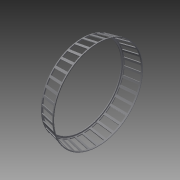
# Autodesk Inventor part: 32912_cage
Saved by Autodesk Inventor 2014 SP2 (Build 180246200, 246)
## iProperties
Created: 2018-11-12
Part Number: 32912_cage
Material: Generic
Catalog Web Link: www.cadenas.de
Description: BT1_001_101_cage-Tapered roller bearings, single row
Vendor: SKF
Document SubType Name: Modeling
Designer: psadmin
Manufacturer: SKF
Mass: 1.044 g
Surface Area: 42.9742 cm^2
Volume: 1.044 cm^3
Density: 1 g/cm^3
Appearance: PSOLRGB-175-175-175
Category: PARTsolutions
Company: SKF
Title: 32912_cage
Author: Cadenas PARTsolutions
Comments: Tapered roller bearings, single row
PSOL_IDENT_0: {$CADENAS_DATA\23d-libs\skf\bearings_units_and_housings\roller_bearings\tapered_roller_bearings\tape
PSOL_IDENT_1: red_roller_bearings_single_row\parts\bt1_001_101_cage.prj},172 {VTYP=3D},{NB=32912_cage},{LINA=32912
PSOL_IDENT_2: _cage},{NN=BT1_001_101_cage},{DATE=14.08.2018 07:35:10},{GEOMDATE=27.06.2018 08:15:48},{VERSION=},{L
PSOL_IDENT_3: INEID=2140},{WBVAR=},{WBNUMERIC=}  {NB=32912_cage},{LINA=32912_cage},{KT=DUMMY},{DESIGNATION=32912},
PSOL_IDENT_4: {DD=60.000},{D=85.000},{T=17.000},{DD1=73.8000},{D1=MIN},{B=17.000},{C=14.000},{C1=MIN},{R12=1.0},{R
PSOL_IDENT_5: 34=1.0},{AA=15.45165},{PITCH=72.347},{DW=5.200},{LW=12.200},{RANGLE=1.600},{ALPHA=12.450},{DDAMAX=67
PSOL_IDENT_6: },{DDAMIN=68.0},{DAMIN=78},{DAMAX=78.0},{DBMIN=81},{CA=3},{CB=3.0},{RA=1.0},{RB=1.0},{LOAD1=53.200},
PSOL_IDENT_7: {LOAD2=75.000},{LOAD3=7.800},{SPEED1=6000},{SPEED2=7000},{EE=0.33},{Y=1.80},{Y0=1.0},{Y1=0},{X1=1},{
PSOL_IDENT_8: X2=0.4},{X0=0.5},{Z=34},{II=1},{R1=0.00000231},{R2=10.9},{S1=0.009},{S2=2},{KZ=6},{KL=0.7},{BF=2},{M
PSOL_IDENT_9: ASS=0.302},{PIM=PIM_BT1_001},{DESIGN=trb1},{HELP=0.000}
NN: BT1_001_101_cage
NT: Tapered roller bearings, single row
NB: 32912_cage
NBSYN: $DESIGNATION._cage
LINA: 32912_cage
DESIGNATION: 32912
DD: 60
D: 85
T: 17
DD1: 73.8
D1: 0
B: 17
C: 14
C1: 0
R12: 1
R34: 1
AA: 15.45165
PITCH: 72.347
DW: 5.2
LW: 12.2
RANGLE: 1.6
ALPHA: 12.45
DDAMAX: 67
DDAMIN: 68
DAMIN: 78
DAMAX: 78
DBMIN: 81
CA: 3
CB: 3
RA: 1
RB: 1
LOAD1: 53.2
LOAD2: 75
LOAD3: 7.8
SPEED1: 6000
SPEED2: 7000
EE: 0.33
Y: 1.8
Y0: 1
Y1: 0
X1: 1
X2: 0.4
X0: 0.5
Z: 34
II: 1
R1: 0.00000231
R2: 10.9
S1: 0.009
S2: 2
KZ: 6
KL: 0.7
BF: 2
MASS: 0.302
PIM: PIM_BT1_001
SUPPLIER: SKF
ARTICLENO: 32912_cage
BOMINFO: 32912_cage
CREATOR: CADENAS GmbH
Autodesk Inventor part; units mm, degrees
sketch "Sketch_1" plane through (0, 0, 0) normal (0, 0, 1) x (1, 0, 0)
  line L0 (0.4926, 0) -> (-0.1574, 0)
  line L1 (-0.1574, 35.8569) -> (-0.1574, 34.6341)
  line L2 (-0.1574, 34.6341) -> (0.4926, 34.6341)
  line L3 (0.4926, 34.6341) -> (0.4926, 35.8569)
  line L4 (0.4926, 35.8569) -> (14.411, 39.0383)
  line L5 (14.411, 39.0383) -> (14.2709, 39.673)
  line L6 (14.2709, 39.673) -> (0.3477, 36.4905)
  arc A0 (0.3477, 36.4905) -> (-0.1574, 35.8569) centre (0.4926, 35.8569) ccw
  constraints: 14 end point, 2 point on circle, 1 centre point
revolve "Revolution1" add sketch "Sketch_1" angle 360 about axis through (0.4926, 0, 0) along (1, 0, 0)
sketch "Sketch_2" plane through (7.1783, 0, 0) normal (1, 0, 0) x (0, 0, -1)
  line L0 (-41.4536, 1.0487) -> (-18.081, 0.4574)
  arc A0 (-18.081, 0.4574) -> (-18.081, -0.4574) centre (0, 0) ccw
  line L1 (-18.081, -0.4574) -> (-41.4536, -1.0487)
  line L2 (-41.4536, -1.0487) -> (-40.9404, -6.5862)
  line L3 (-40.9404, -6.5862) -> (-17.8572, -2.8727)
  arc A1 (-17.8572, -2.8727) -> (-17.6891, -3.772) centre (0, 0) ccw
  line L4 (-17.6891, -3.772) -> (-40.555, -8.6479)
  line L5 (-40.555, -8.6479) -> (-39.0331, -13.9969)
  line L6 (-39.0331, -13.9969) -> (-17.0252, -6.1051)
  arc A2 (-17.0252, -6.1051) -> (-16.6948, -6.9581) centre (0, 0) ccw
  line L7 (-16.6948, -6.9581) -> (-38.2755, -15.9527)
  line L8 (-38.2755, -15.9527) -> (-35.7966, -20.9309)
  line L9 (-35.7966, -20.9309) -> (-15.6135, -9.1295)
  arc A3 (-15.6135, -9.1295) -> (-15.1319, -9.9073) centre (0, 0) ccw
  line L10 (-15.1319, -9.9073) -> (-34.6925, -22.7141)
  line L11 (-34.6925, -22.7141) -> (-31.3411, -27.1521)
  line L12 (-31.3411, -27.1521) -> (-13.6702, -11.843)
  arc A4 (-13.6702, -11.843) -> (-13.0538, -12.5191) centre (0, 0) ccw
  line L13 (-13.0538, -12.5191) -> (-29.928, -28.7021)
  line L14 (-29.928, -28.7021) -> (-25.8183, -32.4487)
  line L15 (-25.8183, -32.4487) -> (-11.2612, -14.1533)
  arc A5 (-11.2612, -14.1533) -> (-10.5312, -14.7046) centre (0, 0) ccw
  line L16 (-10.5312, -14.7046) -> (-24.1445, -33.7127)
  line L17 (-24.1445, -33.7127) -> (-19.4162, -36.6403)
  line L18 (-19.4162, -36.6403) -> (-8.4688, -15.9815)
  arc A6 (-8.4688, -15.9815) -> (-7.6499, -16.3893) centre (0, 0) ccw
  line L19 (-7.6499, -16.3893) -> (-17.5387, -37.5752)
  line L20 (-17.5387, -37.5752) -> (-12.353, -39.5841)
  line L21 (-12.353, -39.5841) -> (-5.3881, -17.2656)
  arc A7 (-5.3881, -17.2656) -> (-4.5081, -17.5159) centre (0, 0) ccw
  line L22 (-4.5081, -17.5159) -> (-10.3356, -40.1581)
  line L23 (-10.3356, -40.1581) -> (-4.8691, -41.18)
  line L24 (-4.8691, -41.18) -> (-2.1238, -17.9616)
  arc A8 (-2.1238, -17.9616) -> (-1.2128, -18.046) centre (0, 0) ccw
  line L25 (-1.2128, -18.046) -> (-2.7806, -41.3735)
  line L26 (-2.7806, -41.3735) -> (2.7806, -41.3735)
  line L27 (2.7806, -41.3735) -> (1.2128, -18.046)
  arc A9 (1.2128, -18.046) -> (2.1238, -17.9616) centre (0, 0) ccw
  line L28 (2.1238, -17.9616) -> (4.8691, -41.18)
  line L29 (4.8691, -41.18) -> (10.3356, -40.1581)
  line L30 (10.3356, -40.1581) -> (4.5081, -17.5159)
  arc A10 (4.5081, -17.5159) -> (5.3881, -17.2656) centre (0, 0) ccw
  line L31 (5.3881, -17.2656) -> (12.353, -39.5841)
  line L32 (12.353, -39.5841) -> (17.5387, -37.5752)
  line L33 (17.5387, -37.5752) -> (7.6499, -16.3893)
  arc A11 (7.6499, -16.3893) -> (8.4688, -15.9815) centre (0, 0) ccw
  line L34 (8.4688, -15.9815) -> (19.4162, -36.6403)
  line L35 (19.4162, -36.6403) -> (24.1445, -33.7127)
  line L36 (24.1445, -33.7127) -> (10.5312, -14.7046)
  arc A12 (10.5312, -14.7046) -> (11.2612, -14.1533) centre (0, 0) ccw
  line L37 (11.2612, -14.1533) -> (25.8183, -32.4487)
  line L38 (25.8183, -32.4487) -> (29.928, -28.7021)
  line L39 (29.928, -28.7021) -> (13.0538, -12.5191)
  arc A13 (13.0538, -12.5191) -> (13.6702, -11.843) centre (0, 0) ccw
  line L40 (13.6702, -11.843) -> (31.3411, -27.1521)
  line L41 (31.3411, -27.1521) -> (34.6925, -22.7141)
  line L42 (34.6925, -22.7141) -> (15.1319, -9.9073)
  arc A14 (15.1319, -9.9073) -> (15.6135, -9.1295) centre (0, 0) ccw
  line L43 (15.6135, -9.1295) -> (35.7966, -20.9309)
  line L44 (35.7966, -20.9309) -> (38.2755, -15.9527)
  line L45 (38.2755, -15.9527) -> (16.6948, -6.9581)
  arc A15 (16.6948, -6.9581) -> (17.0252, -6.1051) centre (0, 0) ccw
  line L46 (17.0252, -6.1051) -> (39.0331, -13.9969)
  line L47 (39.0331, -13.9969) -> (40.555, -8.6479)
  line L48 (40.555, -8.6479) -> (17.6891, -3.772)
  arc A16 (17.6891, -3.772) -> (17.8572, -2.8727) centre (0, 0) ccw
  line L49 (17.8572, -2.8727) -> (40.9404, -6.5862)
  line L50 (40.9404, -6.5862) -> (41.4536, -1.0487)
  line L51 (41.4536, -1.0487) -> (18.081, -0.4574)
  arc A17 (18.081, -0.4574) -> (18.081, 0.4574) centre (0, 0) ccw
  line L52 (18.081, 0.4574) -> (41.4536, 1.0487)
  line L53 (41.4536, 1.0487) -> (40.9404, 6.5862)
  line L54 (40.9404, 6.5862) -> (17.8572, 2.8727)
  arc A18 (17.8572, 2.8727) -> (17.6891, 3.772) centre (0, 0) ccw
  line L55 (17.6891, 3.772) -> (40.555, 8.6479)
  line L56 (40.555, 8.6479) -> (39.0331, 13.9969)
  line L57 (39.0331, 13.9969) -> (17.0252, 6.1051)
  arc A19 (17.0252, 6.1051) -> (16.6948, 6.9581) centre (0, 0) ccw
  line L58 (16.6948, 6.9581) -> (38.2755, 15.9527)
  line L59 (38.2755, 15.9527) -> (35.7966, 20.9309)
  line L60 (35.7966, 20.9309) -> (15.6135, 9.1295)
  arc A20 (15.6135, 9.1295) -> (15.1319, 9.9073) centre (0, 0) ccw
  line L61 (15.1319, 9.9073) -> (34.6925, 22.7141)
  line L62 (34.6925, 22.7141) -> (31.3411, 27.1521)
  line L63 (31.3411, 27.1521) -> (13.6702, 11.843)
  arc A21 (13.6702, 11.843) -> (13.0538, 12.5191) centre (0, 0) ccw
  line L64 (13.0538, 12.5191) -> (29.928, 28.7021)
  line L65 (29.928, 28.7021) -> (25.8183, 32.4487)
  line L66 (25.8183, 32.4487) -> (11.2612, 14.1533)
  arc A22 (11.2612, 14.1533) -> (10.5312, 14.7046) centre (0, 0) ccw
  line L67 (10.5312, 14.7046) -> (24.1445, 33.7127)
  line L68 (24.1445, 33.7127) -> (19.4162, 36.6403)
  line L69 (19.4162, 36.6403) -> (8.4688, 15.9815)
  arc A23 (8.4688, 15.9815) -> (7.6499, 16.3893) centre (0, 0) ccw
  line L70 (7.6499, 16.3893) -> (17.5387, 37.5752)
  line L71 (17.5387, 37.5752) -> (12.353, 39.5841)
  line L72 (12.353, 39.5841) -> (5.3881, 17.2656)
  arc A24 (5.3881, 17.2656) -> (4.5081, 17.5159) centre (0, 0) ccw
  line L73 (4.5081, 17.5159) -> (10.3356, 40.1581)
  line L74 (10.3356, 40.1581) -> (4.8691, 41.18)
  line L75 (4.8691, 41.18) -> (2.1238, 17.9616)
  arc A25 (2.1238, 17.9616) -> (1.2128, 18.046) centre (0, 0) ccw
  line L76 (1.2128, 18.046) -> (2.7806, 41.3735)
  line L77 (2.7806, 41.3735) -> (-2.7806, 41.3735)
  line L78 (-2.7806, 41.3735) -> (-1.2128, 18.046)
  arc A26 (-1.2128, 18.046) -> (-2.1238, 17.9616) centre (0, 0) ccw
  line L79 (-2.1238, 17.9616) -> (-4.8691, 41.18)
  line L80 (-4.8691, 41.18) -> (-10.3356, 40.1581)
  line L81 (-10.3356, 40.1581) -> (-4.5081, 17.5159)
  arc A27 (-4.5081, 17.5159) -> (-5.3881, 17.2656) centre (0, 0) ccw
  line L82 (-5.3881, 17.2656) -> (-12.353, 39.5841)
  line L83 (-12.353, 39.5841) -> (-17.5387, 37.5752)
  line L84 (-17.5387, 37.5752) -> (-7.6499, 16.3893)
  arc A28 (-7.6499, 16.3893) -> (-8.4688, 15.9815) centre (0, 0) ccw
  line L85 (-8.4688, 15.9815) -> (-19.4162, 36.6403)
  line L86 (-19.4162, 36.6403) -> (-24.1445, 33.7127)
  line L87 (-24.1445, 33.7127) -> (-10.5312, 14.7046)
  arc A29 (-10.5312, 14.7046) -> (-11.2612, 14.1533) centre (0, 0) ccw
  line L88 (-11.2612, 14.1533) -> (-25.8183, 32.4487)
  line L89 (-25.8183, 32.4487) -> (-29.928, 28.7021)
  line L90 (-29.928, 28.7021) -> (-13.0538, 12.5191)
  arc A30 (-13.0538, 12.5191) -> (-13.6702, 11.843) centre (0, 0) ccw
  line L91 (-13.6702, 11.843) -> (-31.3411, 27.1521)
  line L92 (-31.3411, 27.1521) -> (-34.6925, 22.7141)
  line L93 (-34.6925, 22.7141) -> (-15.1319, 9.9073)
  arc A31 (-15.1319, 9.9073) -> (-15.6135, 9.1295) centre (0, 0) ccw
  line L94 (-15.6135, 9.1295) -> (-35.7966, 20.9309)
  line L95 (-35.7966, 20.9309) -> (-38.2755, 15.9527)
  line L96 (-38.2755, 15.9527) -> (-16.6948, 6.9581)
  arc A32 (-16.6948, 6.9581) -> (-17.0252, 6.1051) centre (0, 0) ccw
  line L97 (-17.0252, 6.1051) -> (-39.0331, 13.9969)
  line L98 (-39.0331, 13.9969) -> (-40.555, 8.6479)
  line L99 (-40.555, 8.6479) -> (-17.6891, 3.772)
  arc A33 (-17.6891, 3.772) -> (-17.8572, 2.8727) centre (0, 0) ccw
  line L100 (-17.8572, 2.8727) -> (-40.9404, 6.5862)
  line L101 (-40.9404, 6.5862) -> (-41.4536, 1.0487)
  constraints: 204 end point, 68 point on circle, 34 centre point
extrude "Extrusion1" cut sketch "Sketch_2" along normal mid plane 12.19
ref_plane "cage_XY" through (0, 0, 0) normal (0, 0, 1) x (1, 0, 0)
ref_plane "cage_YZ" through (0, 0, 0) normal (1, 0, 0) x (0, 1, 0)
ref_plane "cage_ZX" through (0, 0, 0) normal (0, 1, 0) x (0, 0, 1)
ref_plane "roller1_XY" through (0, 36.1735, 0) normal (1, 0, 0) x (0, 0, -1)
ref_plane "roller1_YZ" through (0, 36.1735, 0) normal (0, 0, -1) x (0, 1, 0)
ref_plane "roller1_ZX" through (0, 36.1735, 0) normal (0, 1, 0) x (1, 0, 0)
ref_plane "roller10_XY" through (0, -3.3377, 36.0192) normal (1, 0, 0) x (0, 0.9957, 0.0923)
ref_plane "roller10_YZ" through (0, -3.3377, 36.0192) normal (0, 0.9957, 0.0923) x (0, -0.0923, 0.9957)
ref_plane "roller10_ZX" through (0, -3.3377, 36.0192) normal (0, -0.0923, 0.9957) x (1, 0, 0)
ref_plane "roller11_XY" through (0, -9.8993, 34.7926) normal (1, 0, 0) x (0, 0.9618, 0.2737)
ref_plane "roller11_YZ" through (0, -9.8993, 34.7926) normal (0, 0.9618, 0.2737) x (0, -0.2737, 0.9618)
ref_plane "roller11_ZX" through (0, -9.8993, 34.7926) normal (0, -0.2737, 0.9618) x (1, 0, 0)
ref_plane "roller12_XY" through (0, -16.1239, 32.3812) normal (1, 0, 0) x (0, 0.8952, 0.4457)
ref_plane "roller12_YZ" through (0, -16.1239, 32.3812) normal (0, 0.8952, 0.4457) x (0, -0.4457, 0.8952)
ref_plane "roller12_ZX" through (0, -16.1239, 32.3812) normal (0, -0.4457, 0.8952) x (1, 0, 0)
ref_plane "roller13_XY" through (0, -21.7994, 28.8671) normal (1, 0, 0) x (0, 0.798, 0.6026)
ref_plane "roller13_YZ" through (0, -21.7994, 28.8671) normal (0, 0.798, 0.6026) x (0, -0.6026, 0.798)
ref_plane "roller13_ZX" through (0, -21.7994, 28.8671) normal (0, -0.6026, 0.798) x (1, 0, 0)
ref_plane "roller14_XY" through (0, -26.7325, 24.3699) normal (1, 0, 0) x (0, 0.6737, 0.739)
ref_plane "roller14_YZ" through (0, -26.7325, 24.3699) normal (0, 0.6737, 0.739) x (0, -0.739, 0.6737)
ref_plane "roller14_ZX" through (0, -26.7325, 24.3699) normal (0, -0.739, 0.6737) x (1, 0, 0)
ref_plane "roller15_XY" through (0, -30.7553, 19.0429) normal (1, 0, 0) x (0, 0.5264, 0.8502)
ref_plane "roller15_YZ" through (0, -30.7553, 19.0429) normal (0, 0.5264, 0.8502) x (0, -0.8502, 0.5264)
ref_plane "roller15_ZX" through (0, -30.7553, 19.0429) normal (0, -0.8502, 0.5264) x (1, 0, 0)
ref_plane "roller16_XY" through (0, -33.7308, 13.0674) normal (1, 0, 0) x (0, 0.3612, 0.9325)
ref_plane "roller16_YZ" through (0, -33.7308, 13.0674) normal (0, 0.3612, 0.9325) x (0, -0.9325, 0.3612)
ref_plane "roller16_ZX" through (0, -33.7308, 13.0674) normal (0, -0.9325, 0.3612) x (1, 0, 0)
ref_plane "roller17_XY" through (0, -35.5576, 6.6469) normal (1, 0, 0) x (0, 0.1837, 0.983)
ref_plane "roller17_YZ" through (0, -35.5576, 6.6469) normal (0, 0.1837, 0.983) x (0, -0.983, 0.1837)
ref_plane "roller17_ZX" through (0, -35.5576, 6.6469) normal (0, -0.983, 0.1837) x (1, 0, 0)
ref_plane "roller18_XY" through (0, -36.1735, 0) normal (1, 0, 0) x (0, 0, 1)
ref_plane "roller18_YZ" through (0, -36.1735, 0) normal (0, 0, 1) x (0, -1, 0)
ref_plane "roller18_ZX" through (0, -36.1735, 0) normal (0, -1, 0) x (1, 0, 0)
ref_plane "roller19_XY" through (0, -35.5576, -6.6469) normal (1, 0, 0) x (0, -0.1837, 0.983)
ref_plane "roller19_YZ" through (0, -35.5576, -6.6469) normal (0, -0.1837, 0.983) x (0, -0.983, -0.1837)
ref_plane "roller19_ZX" through (0, -35.5576, -6.6469) normal (0, -0.983, -0.1837) x (1, 0, 0)
ref_plane "roller2_XY" through (0, 35.5576, 6.6469) normal (1, 0, 0) x (0, 0.1837, -0.983)
ref_plane "roller2_YZ" through (0, 35.5576, 6.6469) normal (0, 0.1837, -0.983) x (0, 0.983, 0.1837)
ref_plane "roller2_ZX" through (0, 35.5576, 6.6469) normal (0, 0.983, 0.1837) x (1, 0, 0)
ref_plane "roller20_XY" through (0, -33.7308, -13.0674) normal (1, 0, 0) x (0, -0.3612, 0.9325)
ref_plane "roller20_YZ" through (0, -33.7308, -13.0674) normal (0, -0.3612, 0.9325) x (0, -0.9325, -0.3612)
ref_plane "roller20_ZX" through (0, -33.7308, -13.0674) normal (0, -0.9325, -0.3612) x (1, 0, 0)
ref_plane "roller21_XY" through (0, -30.7553, -19.0429) normal (1, 0, 0) x (0, -0.5264, 0.8502)
ref_plane "roller21_YZ" through (0, -30.7553, -19.0429) normal (0, -0.5264, 0.8502) x (0, -0.8502, -0.5264)
ref_plane "roller21_ZX" through (0, -30.7553, -19.0429) normal (0, -0.8502, -0.5264) x (1, 0, 0)
ref_plane "roller22_XY" through (0, -26.7325, -24.3699) normal (1, 0, 0) x (0, -0.6737, 0.739)
ref_plane "roller22_YZ" through (0, -26.7325, -24.3699) normal (0, -0.6737, 0.739) x (0, -0.739, -0.6737)
ref_plane "roller22_ZX" through (0, -26.7325, -24.3699) normal (0, -0.739, -0.6737) x (1, 0, 0)
ref_plane "roller23_XY" through (0, -21.7994, -28.8671) normal (1, 0, 0) x (0, -0.798, 0.6026)
ref_plane "roller23_YZ" through (0, -21.7994, -28.8671) normal (0, -0.798, 0.6026) x (0, -0.6026, -0.798)
ref_plane "roller23_ZX" through (0, -21.7994, -28.8671) normal (0, -0.6026, -0.798) x (1, 0, 0)
ref_plane "roller24_XY" through (0, -16.1239, -32.3812) normal (1, 0, 0) x (0, -0.8952, 0.4457)
ref_plane "roller24_YZ" through (0, -16.1239, -32.3812) normal (0, -0.8952, 0.4457) x (0, -0.4457, -0.8952)
ref_plane "roller24_ZX" through (0, -16.1239, -32.3812) normal (0, -0.4457, -0.8952) x (1, 0, 0)
ref_plane "roller25_XY" through (0, -9.8993, -34.7926) normal (1, 0, 0) x (0, -0.9618, 0.2737)
ref_plane "roller25_YZ" through (0, -9.8993, -34.7926) normal (0, -0.9618, 0.2737) x (0, -0.2737, -0.9618)
ref_plane "roller25_ZX" through (0, -9.8993, -34.7926) normal (0, -0.2737, -0.9618) x (1, 0, 0)
ref_plane "roller26_XY" through (0, -3.3377, -36.0192) normal (1, 0, 0) x (0, -0.9957, 0.0923)
ref_plane "roller26_YZ" through (0, -3.3377, -36.0192) normal (0, -0.9957, 0.0923) x (0, -0.0923, -0.9957)
ref_plane "roller26_ZX" through (0, -3.3377, -36.0192) normal (0, -0.0923, -0.9957) x (1, 0, 0)
ref_plane "roller27_XY" through (0, 3.3377, -36.0192) normal (1, 0, 0) x (0, -0.9957, -0.0923)
ref_plane "roller27_YZ" through (0, 3.3377, -36.0192) normal (0, -0.9957, -0.0923) x (0, 0.0923, -0.9957)
ref_plane "roller27_ZX" through (0, 3.3377, -36.0192) normal (0, 0.0923, -0.9957) x (1, 0, 0)
ref_plane "roller28_XY" through (0, 9.8993, -34.7926) normal (1, 0, 0) x (0, -0.9618, -0.2737)
ref_plane "roller28_YZ" through (0, 9.8993, -34.7926) normal (0, -0.9618, -0.2737) x (0, 0.2737, -0.9618)
ref_plane "roller28_ZX" through (0, 9.8993, -34.7926) normal (0, 0.2737, -0.9618) x (1, 0, 0)
ref_plane "roller29_XY" through (0, 16.1239, -32.3812) normal (1, 0, 0) x (0, -0.8952, -0.4457)
ref_plane "roller29_YZ" through (0, 16.1239, -32.3812) normal (0, -0.8952, -0.4457) x (0, 0.4457, -0.8952)
ref_plane "roller29_ZX" through (0, 16.1239, -32.3812) normal (0, 0.4457, -0.8952) x (1, 0, 0)
ref_plane "roller3_XY" through (0, 33.7308, 13.0674) normal (1, 0, 0) x (0, 0.3612, -0.9325)
ref_plane "roller3_YZ" through (0, 33.7308, 13.0674) normal (0, 0.3612, -0.9325) x (0, 0.9325, 0.3612)
ref_plane "roller3_ZX" through (0, 33.7308, 13.0674) normal (0, 0.9325, 0.3612) x (1, 0, 0)
ref_plane "roller30_XY" through (0, 21.7994, -28.8671) normal (1, 0, 0) x (0, -0.798, -0.6026)
ref_plane "roller30_YZ" through (0, 21.7994, -28.8671) normal (0, -0.798, -0.6026) x (0, 0.6026, -0.798)
ref_plane "roller30_ZX" through (0, 21.7994, -28.8671) normal (0, 0.6026, -0.798) x (1, 0, 0)
ref_plane "roller31_XY" through (0, 26.7325, -24.3699) normal (1, 0, 0) x (0, -0.6737, -0.739)
ref_plane "roller31_YZ" through (0, 26.7325, -24.3699) normal (0, -0.6737, -0.739) x (0, 0.739, -0.6737)
ref_plane "roller31_ZX" through (0, 26.7325, -24.3699) normal (0, 0.739, -0.6737) x (1, 0, 0)
ref_plane "roller32_XY" through (0, 30.7553, -19.0429) normal (1, 0, 0) x (0, -0.5264, -0.8502)
ref_plane "roller32_YZ" through (0, 30.7553, -19.0429) normal (0, -0.5264, -0.8502) x (0, 0.8502, -0.5264)
ref_plane "roller32_ZX" through (0, 30.7553, -19.0429) normal (0, 0.8502, -0.5264) x (1, 0, 0)
ref_plane "roller33_XY" through (0, 33.7308, -13.0674) normal (1, 0, 0) x (0, -0.3612, -0.9325)
ref_plane "roller33_YZ" through (0, 33.7308, -13.0674) normal (0, -0.3612, -0.9325) x (0, 0.9325, -0.3612)
ref_plane "roller33_ZX" through (0, 33.7308, -13.0674) normal (0, 0.9325, -0.3612) x (1, 0, 0)
ref_plane "roller34_XY" through (0, 35.5576, -6.6469) normal (1, 0, 0) x (0, -0.1837, -0.983)
ref_plane "roller34_YZ" through (0, 35.5576, -6.6469) normal (0, -0.1837, -0.983) x (0, 0.983, -0.1837)
ref_plane "roller34_ZX" through (0, 35.5576, -6.6469) normal (0, 0.983, -0.1837) x (1, 0, 0)
ref_plane "roller4_XY" through (0, 30.7553, 19.0429) normal (1, 0, 0) x (0, 0.5264, -0.8502)
ref_plane "roller4_YZ" through (0, 30.7553, 19.0429) normal (0, 0.5264, -0.8502) x (0, 0.8502, 0.5264)
ref_plane "roller4_ZX" through (0, 30.7553, 19.0429) normal (0, 0.8502, 0.5264) x (1, 0, 0)
ref_plane "roller5_XY" through (0, 26.7325, 24.3699) normal (1, 0, 0) x (0, 0.6737, -0.739)
ref_plane "roller5_YZ" through (0, 26.7325, 24.3699) normal (0, 0.6737, -0.739) x (0, 0.739, 0.6737)
ref_plane "roller5_ZX" through (0, 26.7325, 24.3699) normal (0, 0.739, 0.6737) x (1, 0, 0)
ref_plane "roller6_XY" through (0, 21.7994, 28.8671) normal (1, 0, 0) x (0, 0.798, -0.6026)
ref_plane "roller6_YZ" through (0, 21.7994, 28.8671) normal (0, 0.798, -0.6026) x (0, 0.6026, 0.798)
ref_plane "roller6_ZX" through (0, 21.7994, 28.8671) normal (0, 0.6026, 0.798) x (1, 0, 0)
ref_plane "roller7_XY" through (0, 16.1239, 32.3812) normal (1, 0, 0) x (0, 0.8952, -0.4457)
ref_plane "roller7_YZ" through (0, 16.1239, 32.3812) normal (0, 0.8952, -0.4457) x (0, 0.4457, 0.8952)
ref_plane "roller7_ZX" through (0, 16.1239, 32.3812) normal (0, 0.4457, 0.8952) x (1, 0, 0)
ref_plane "roller8_XY" through (0, 9.8993, 34.7926) normal (1, 0, 0) x (0, 0.9618, -0.2737)
ref_plane "roller8_YZ" through (0, 9.8993, 34.7926) normal (0, 0.9618, -0.2737) x (0, 0.2737, 0.9618)
ref_plane "roller8_ZX" through (0, 9.8993, 34.7926) normal (0, 0.2737, 0.9618) x (1, 0, 0)
ref_plane "roller9_XY" through (0, 3.3377, 36.0192) normal (1, 0, 0) x (0, 0.9957, -0.0923)
ref_plane "roller9_YZ" through (0, 3.3377, 36.0192) normal (0, 0.9957, -0.0923) x (0, 0.0923, 0.9957)
ref_plane "roller9_ZX" through (0, 3.3377, 36.0192) normal (0, 0.0923, 0.9957) x (1, 0, 0)
body "Solid1"
